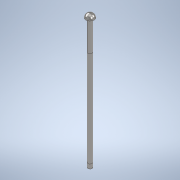
# Autodesk Inventor part: Haste Contrapeso
Saved by Autodesk Inventor 2021 (Build 250183000, 183)
## iProperties
Created: 2021-08-26
Part Number: Haste Contrapeso
Material: Steel, Carbon
Document SubType Name: Modeling
Designer: guilh
Density: 7.85 g/cm^3
Appearance: Semi-Polished
Mass: 1635.88 g
Surface Area: 420.973 cm^2
Volume: 208.392 cm^3
Author: guilh
Autodesk Inventor part; units mm, degrees
ref_plane "YZ Plane" through (0, 0, 0) normal (1, 0, 0) x (0, 1, 0)
ref_plane "XZ Plane" through (0, 0, 0) normal (0, 1, 0) x (-1, 0, 0)
ref_plane "XY Plane" through (0, 0, 0) normal (0, 0, 1) x (1, 0, 0)
sketch "Sketch1" plane through (0, 0, 0) normal (0, 1, 0) x (-1, 0, 0)
  circle A0 centre (0, 0) radius 10
  dimension "d0" = 20
  constraints: 1 centre point, 1 coincident
  measures "d0" diameter of A0
extrude "Extrusion1" add sketch "Sketch1" along normal blind 610
sketch "Sketch2" plane through (0, 610, 0) normal (0, 1, 0) x (1, 0, 0)
  circle A0 centre (0, 0) radius 20
  dimension "d3" = 40
  constraints: 1 centre point, 1 coincident
  measures "d3" diameter of A0
extrude "Extrusion2" add sketch "Sketch2" along normal blind 20
fillet "Fillet1" radius 20 1 edges at (-20, 630, 0)
sketch "Sketch3" plane through (0, 0, 0) normal (0, 0, 1) x (1, 0, 0)
  line L0 (20, 610) -> (-20, 610) projected
  line L1 (-20, 610) -> (20, 610)
  line L2 (20, 610) -> (20, 469.6128)
  line L3 (20, 469.6128) -> (-20, 469.6128)
  line L4 (-20, 469.6128) -> (-20, 610)
  point P0 (0, 0)
  constraints: 8 end point, 3 perpendicular, 1 horizontal
split_face "Split1"
sketch "Sketch4" plane through (0, 0, 0) normal (0, 0, 1) x (1, 0, 0)
  line L0 (0, 0) -> (27.9883, 0)
  line L1 (27.9883, 0) -> (27.9883, 20.3959)
  line L2 (27.9883, 20.3959) -> (-23.698, 20.3959)
  line L3 (-23.698, 20.3959) -> (-23.698, 0)
  line L4 (-23.698, 0) -> (27.9883, 0)
  constraints: 10 end point, 3 perpendicular, 1 collinear, 1 horizontal, 1 point on line
split_face "Split2"
sketch "Sketch5" plane through (0, 0, 0) normal (0, 0, 1) x (1, 0, 0)
  line L0 (10, 469.6128) -> (-10, 469.6128) projected
  line L1 (-6.0106, 469.6128) -> (-6.0106, 612.6424)
  line L2 (-6.0106, 612.6424) -> (-55.0341, 605.0239)
  line L3 (-55.0341, 605.0239) -> (-35.491, 440.7287)
  line L4 (-35.491, 440.7287) -> (-6.0106, 469.6128)
  point P0 (0, 0)
  constraints: 8 end point, 1 point on line, 1 vertical
split_face "Split3"
body "Solid1"
